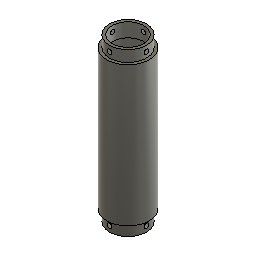
Link_250mm (Autodesk Fusion 360 design; units mm, degrees)
part number: 2025-04-26-16-47-43-513
Autodesk Fusion 360 part; units mm, degrees
sketch "Sketch1" plane through (0, 0, 0) normal (0, 1, 0) x (1, 0, 0)
  circle A0 centre (0, 0) radius 33.1
  circle A1 centre (0, 0) radius 28.1
  dimension "d1" = 66.2
  dimension "d2" = 5
  constraint coincident A0.centre A1.centre
  constraint concentric A0 A1
  measures "d1" diameter of A0
  measures "d2" distance of A0 A1
extrude "Extrude1" add sketch "Sketch1" along normal blind 25
sketch "Sketch2" plane through (0, 0, 0) normal (0, 1, 0) x (1, 0, 0)
  circle A0 centre (0, 0) radius 33.1
  circle A1 centre (0, 0) radius 38.1
  dimension "d5" = 66.2
  dimension "d6" = 5
  constraint coincident A0.centre A1.centre
  constraint concentric A0 A1
  measures "d5" diameter of A0
  measures "d6" distance of A0 A1
extrude "Extrude2" add sketch "Sketch2" along normal blind 250 from surface at 20
sketch "Sketch3" plane through (0, 270, 0) normal (0, 1, 0) x (-1, 0, 0)
  circle A0 centre (0, 0) radius 33.1
  circle A1 centre (0, 0) radius 38.1
  circle A2 centre (0, 0) radius 33.1
  circle A3 centre (0, 0) radius 28.1
  dimension "d10" = 66.2
  dimension "d11" = 5
  constraint coincident A0.centre A1.centre
  measures "d10" diameter of A2
  measures "d11" distance of A2 A3
extrude "Extrude3" add sketch "Sketch3" along normal blind 25 from surface at -5 contours A0 A2
sketch "Sketch4" plane through (0, 0, 0) normal (0, 0, 1) x (1, 0, 0)
  circle A0 centre (0, 10) radius 4
  circle A1 centre (0, 280) radius 4
  line L0 (33.1, 290) -> (-33.1, 290)
  dimension "d15" = 8
  dimension "d16" = 10
  dimension "d17" = 8
  dimension "d18" = 10
  measures "d15" diameter of A0
  measures "d16" distance of origin A0.centre
  measures "d17" diameter of A1
  measures "d18" distance of A1.centre L0
extrude "Extrude4" cut sketch "Sketch4" along normal mid plane 100
sketch "Sketch5" plane through (0, 0, 0) normal (1, 0, 0) x (0, 0, -1)
  circle A0 centre (0, 10) radius 4
  line L0 (33.1, 0) -> (-33.1, 0)
  circle A1 centre (0, 280) radius 4
  line L1 (33.1, 290) -> (-33.1, 290)
  dimension "d21" = 8
  dimension "d22" = 10
  dimension "d23" = 8
  dimension "d24" = 10
  measures "d21" diameter of A0
  measures "d22" distance of A0.centre L0
  measures "d23" diameter of A1
  measures "d24" distance of A1.centre L1
extrude "Extrude5" cut sketch "Sketch5" along normal mid plane 120
equation "d13 = 28 mm - 3 mm"
